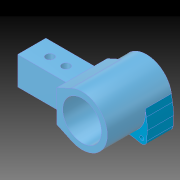
# Autodesk Inventor part: KB33-046-003-001 - Крепление
Saved by Autodesk Inventor 2020 (Build 240168000, 168)
## iProperties
Created: 2021-06-09
Part Number: KB33-046-003-001 - Крепление
Material: ABS Plastic
Document SubType Name: Modeling
Designer: Петров Иван
Density: 1.06 g/cm^3
Appearance: Smooth - Navy
Mass: 107.224 g
Surface Area: 296.859 cm^2
Volume: 101.155 cm^3
Author: Петров Иван
Autodesk Inventor part; units mm, degrees
ref_plane "XZ Plane" through (0, 0, 0) normal (0, 1, 0) x (-1, 0, 0)
ref_plane "XY Plane" through (0, 0, 0) normal (0, 0, 1) x (1, 0, 0)
sketch "Sketch1" plane through (0, 0, 0) normal (0, 0, 1) x (1, 0, 0)
  circle A0 centre (0, 0) radius 19.25
  circle A1 centre (0, 0) radius 25
  dimension "d0" = 38.5
  dimension "d1" = 50
  constraints: 2 centre point, 2 coincident
  measures "d0" diameter of A0
  measures "d1" diameter of A1
extrude "Extrusion1" add sketch "Sketch1" along normal blind 60
sketch "Sketch2" plane through (0, 0, 0) normal (0, 0, -1) x (-1, 0, 0)
  circle A0 centre (0, 0) radius 25
  arc A1 (-2.9173, -11.1238) -> (-11.1238, -2.9173) centre (0, 0) ccw
  arc A2 (-11.1238, -2.9173) -> (-2.9173, -11.1238) centre (-4.9497, -4.9497) ccw
  circle A3 centre (10.6066, -10.6066) radius 1.25
  circle A4 centre (14.4889, 3.8823) radius 1.25
  circle A5 centre (3.8823, 14.4889) radius 1.25
  circle A6 centre (-10.6066, 10.6066) radius 1.25
  circle A7 centre (-14.4889, -3.8823) radius 1.25
  circle A8 centre (-3.8823, -14.4889) radius 1.25
  circle A9 centre (-4.9497, -4.9497) radius 6
  arc A10 (-3.8284, -10.844) -> (-10.844, -3.8284) centre (-4.9497, -4.9497) ccw
  spline S0 degree 3 poles (-10.844, -3.8284) (-10.8607, -3.916) (-10.8757, -4.0054) (-10.8888, -4.0967) knots 0 0 0 0 1 1 1 1
  arc A11 (-10.8888, -4.0967) -> (-4.0967, -10.8888) centre (-4.9497, -4.9497) ccw
  spline S1 degree 3 poles (-4.0967, -10.8888) (-4.0054, -10.8757) (-3.916, -10.8607) (-3.8284, -10.844) knots 0 0 0 0 1 1 1 1
  dimension "d4" = 50
  constraints: 12 centre point, 8 point on circle, 7 other
  measures "d4" diameter of A0
extrude "Extrusion2" add sketch "Sketch2" along normal blind 4 contours A0 | A2 A1
sketch "Sketch3" plane through (0, 0, -4) normal (0, 0, -1) x (-1, 0, 0)
  arc A0 (-3.8284, -10.844) -> (-10.844, -3.8284) centre (-4.9497, -4.9497) ccw projected
  circle A1 centre (-4.9497, -4.9497) radius 6.5
  point P0 (0, 0)
  dimension "d7" = 13
  constraints: 1 centre point, 1 coincident
  measures "d7" diameter of A1
extrude "Extrusion3" cut sketch "Sketch3" against normal blind 4
ref_plane "Work Plane1" through (-25, 0, 0) normal (1, 0, 0) x (0, 1, 0)
sketch "Sketch5" plane through (0, 0, 60) normal (0, 0, 1) x (1, 0, 0)
  circle A0 centre (0, 0) radius 25 projected
  line L0 (-19.2094, -16) -> (-25, -16)
  line L1 (-25, -16) -> (-25, 16)
  line L2 (-25, 16) -> (-19.2094, 16)
  circle A1 centre (0, 0) radius 19.25 projected
  line L3 (-19.2094, 16) -> (-19.2094, 1.25)
  line L4 (-19.2094, -1.25) -> (-19.2094, -16)
  dimension "d84" = 32
  constraints: 10 end point, 4 point on circle, 3 parallel, 1 horizontal, 1 perpendicular, 1 tangent
  measures "d84" distance of L0.end L1.end
extrude "Extrusion4" add sketch "Sketch5" against normal blind 50 contours L3 A1 L4 A0 | A0 L1 L2 | L0 L1 A0 picked at (-20.2622, -9.4719)
fillet "Сопряжение13" radius 386.75 2 edges at (-19.2094, -16, 35) (-19.2094, 16, 35)
sketch "Эскиз26" plane through (-25, -16, 60) normal (-1, 0, 0) x (0, 0, 1)
  line L0 (0, 32) -> (0, 0) projected
  line L1 (0, 32) -> (-50, 32) projected
  line L2 (-50, 16) -> (-50, 32) projected
  line L3 (-50, 0) -> (-50, 16) projected
  line L4 (0, 0) -> (-50, 0) projected
  line L5 (-50, 0) -> (-50, 16) projected
  line L6 (-50, 16) -> (0, 16) construction
  line L7 (0, 35.25) -> (0, -3.25) projected
  line L8 (-11, 2) -> (-39, 2)
  line L9 (-39, 2) -> (-39, 30)
  line L10 (-39, 30) -> (-11, 30)
  line L11 (-11, 30) -> (-11, 2)
  line L12 (-11, 2) -> (-39, 30) construction
  line L13 (-39, 2) -> (-11, 30) construction
  point P0 (-60, 16)
  point P1 (-25, 16)
  dimension "d104" = 28
  dimension "d105" = 28
  constraints: 14 end point, 4 midpoint, 2 parallel, 1 horizontal, 1 perpendicular
  measures "d104" distance of L9.end L10.end
  measures "d105" distance of L8.end L9.end
extrude "Выдавливание18" add sketch "Эскиз26" along normal blind 50 contours L8 L9 L10 L11
sketch "Эскиз27" plane through (-25, -14, 21) normal (0, -1, 0) x (1, 0, 0)
  line L0 (-50, 0) -> (-50, 28) projected
  line L1 (-50, 14) -> (0, 14) construction
  line L2 (0, 39) -> (0, -11) projected
  circle A0 centre (-16, 14) radius 4
  circle A1 centre (-32, 14) radius 4
  point P0 (25, -21)
  dimension "d112" = 8
  dimension "d113" = 16
  dimension "d114" = 8
  dimension "d115" = 16
  constraints: 2 centre point, 2 end point, 2 midpoint, 2 point on line
  measures "d112" diameter of A0
  measures "d113" distance from line of L2 A0.centre
  measures "d114" diameter of A1
  measures "d115" distance of A0.centre A1.centre
extrude "Выдавливание19" cut sketch "Эскиз27" against normal through all
sketch "Эскиз28" plane through (0, 0, -4) normal (0, 0, -1) x (-1, 0, 0)
  circle A0 centre (-4.9497, -4.9497) radius 6.5 projected
  circle A1 centre (-3.8823, -14.4889) radius 1.25 projected
  circle A2 centre (-14.4889, -3.8823) radius 1.25 projected
  circle A3 centre (-10.6066, 10.6066) radius 1.25 projected
  circle A4 centre (3.8823, 14.4889) radius 1.25 projected
  circle A5 centre (14.4889, 3.8823) radius 1.25 projected
  circle A6 centre (10.6066, -10.6066) radius 1.25 projected
  circle A7 centre (0, 0) radius 25 projected
sketch "Эскиз29" plane through (0, 0, -4) normal (0, 0, -1) x (-1, 0, 0)
  circle A0 centre (-21.3052, -23.3889) radius 2 projected
  arc A1 (19.8436, 9.3826) -> (18.8978, 11.1658) centre (0, 0) ccw projected
  line L0 (18.8978, 11.1658) -> (-3.6525, 19.3734) projected
  line L1 (-3.6525, 19.3734) -> (-3.7551, 19.0915) projected
  line L2 (-8.882, 16.7008) -> (-3.7551, 19.0915) projected
  line L3 (-8.882, 16.7008) -> (-12.524, 18.0264) projected
  arc A2 (-12.524, 18.0264) -> (-21.7153, 3.2016) centre (0, 0) ccw projected
  arc A3 (-22.635, -2.7823) -> (-21.7153, 3.2016) centre (-510.4323, 75.2547) ccw projected
  arc A4 (3.2016, -21.7153) -> (-2.7823, -22.635) centre (75.2547, -510.4323) ccw projected
  arc A5 (3.2016, -21.7153) -> (21.5789, -4.0191) centre (0, 0) ccw projected
  line L4 (21.5789, -4.0191) -> (13.567, -1.103) projected
  arc A6 (12.4454, -0.0837) -> (13.567, -1.103) centre (14.251, 0.7764) ccw projected
  line L5 (12.4454, -0.0837) -> (10.1791, 4.6743) projected
  arc A7 (10.3153, 6.6357) -> (10.1791, 4.6743) centre (11.9848, 5.5344) ccw projected
  arc A8 (16.199, 8.5807) -> (10.3153, 6.6357) centre (14.4889, 3.8823) ccw projected
  line L6 (16.199, 8.5807) -> (16.883, 10.4601) projected
  line L7 (19.8436, 9.3826) -> (16.883, 10.4601) projected
  arc A9 (-25.7776, -3.153) -> (-24.7356, 3.6264) centre (-513.5109, 75.2833) ccw projected
  arc A10 (3.6264, -24.7356) -> (-24.7356, 3.6264) centre (0, 0) ccw projected
  arc A11 (3.6264, -24.7356) -> (-3.153, -25.7776) centre (75.2833, -513.5109) ccw projected
  arc A12 (-4.9507, -25.9827) -> (-3.153, -25.7776) centre (-6.2874, -6.2874) ccw projected
  arc A13 (-4.9507, -25.9827) -> (-20.1699, -28.2583) centre (1.516, -121.2635) ccw projected
  arc A14 (-26.3041, -23.4934) -> (-20.1699, -28.2583) centre (-21.3052, -23.3889) ccw projected
  arc A15 (-26.3041, -23.4934) -> (-26.6145, -14.3007) centre (-384.226, -30.9739) ccw projected
  arc A16 (-25.7776, -3.153) -> (-26.6145, -14.3007) centre (19.4459, -12.1532) ccw projected
  circle A17 centre (14.4889, 3.8823) radius 1.25 projected
  circle A18 centre (0, 0) radius 25 projected
extrude "Выдавливание20" add sketch "Эскиз29" against normal blind 26 contours A9 A18 A11 A12 A13 A14 A15 A16
body "Solid1"
